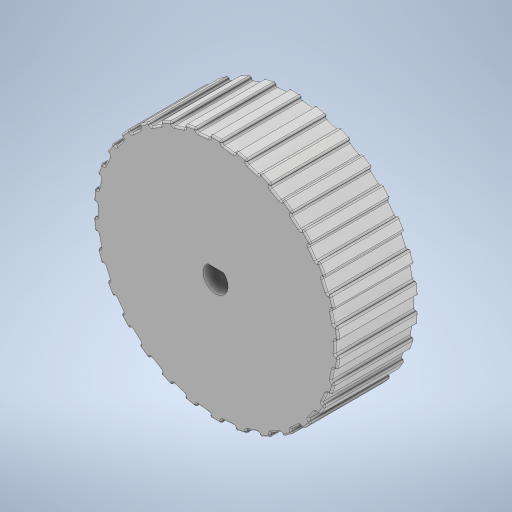
# Autodesk Inventor part: Tyre
Saved by Autodesk Inventor 2024 (Build 280153000, 153)
## iProperties
Created: 2024-04-29
Part Number: Tyre
Material: Generic
Document SubType Name: Modeling
Designer: Hitesh
Density: 1 g/cm^3
Appearance: Default
Author: Hitesh
Autodesk Inventor part; units mm, degrees
ref_plane "YZ Plane" through (0, 0, 0) normal (1, 0, 0) x (0, 1, 0)
ref_plane "XZ Plane" through (0, 0, 0) normal (0, 1, 0) x (-1, 0, 0)
ref_plane "XY Plane" through (0, 0, 0) normal (0, 0, 1) x (1, 0, 0)
sketch "Sketch1" plane through (0, 0, 0) normal (0, 0, 1) x (1, 0, 0)
  circle A0 centre (0, 0) radius 15.2 construction
  circle A1 centre (0, 0) radius 14.75
  circle A2 centre (0, 0) radius 13.5
  spline S0 degree 4 poles (-9.3055, 9.7805) (-7.3263, 12.0552) (-5.2624, 11.3174) (-0.0971, 11.8986) (3.041, 8.7469) (5.0437, 5.9417) (3.2663, 3.137) (1.327, 1.688) knots 0 0 0 0 0 0.374915 0.513644 0.64633 1 1 1 1 1
  circle A3 centre (0, 0) radius 2.1471
  spline S1 degree 4 poles (-11.2034, 7.5322) (-8.1625, 9.7041) (-7.2259, 9.5039) (-2.5238, 11.0895) (1.6832, 7.0671) (2.0649, 4.7541) (1.3, 2.8599) (0, 2.1471) knots 0 0 0 0 0 0.401494 0.546116 0.685045 1 1 1 1 1
  spline S2 degree 4 poles (-13.2771, 2.4429) (-13.0129, 5.4466) (-10.9095, 6.0628) (-7.0724, 9.5691) (-2.6811, 8.8638) (0.588, 7.7715) (0.7987, 4.4578) (0.0814, 2.1456) knots 0 0 0 0 0 0.374915 0.513644 0.64633 1 1 1 1 1
  spline S3 degree 4 poles (-13.4911, -0.4915) (-12.3075, 3.053) (-11.4322, 3.4416) (-8.5601, 7.4882) (-2.7922, 6.7067) (-1.1238, 5.0599) (-0.6293, 3.0778) (-1.2621, 1.7371) knots 0 0 0 0 0 0.401494 0.546116 0.685045 1 1 1 1 1
  spline S4 degree 4 poles (-12.1773, -5.8277) (-13.7291, -3.2424) (-12.3896, -1.5076) (-11.3462, 3.5845) (-7.3791, 5.5951) (-4.0923, 6.6329) (-1.9741, 4.0759) (-1.1953, 1.7837) knots 0 0 0 0 0 0.374915 0.513644 0.64633 1 1 1 1 1
  spline S5 degree 4 poles (-10.6256, -8.3274) (-11.7515, -4.7642) (-11.2717, -3.9354) (-11.3267, 1.0266) (-6.2011, 3.7846) (-3.8833, 3.433) (-2.3182, 2.1201) (-2.0421, 0.6635) knots 0 0 0 0 0 0.401494 0.546116 0.685045 1 1 1 1 1
  spline S6 degree 4 poles (-6.4262, -11.8724) (-9.2012, -10.693) (-9.1373, -8.5021) (-11.2862, -3.7692) (-9.2585, 0.1892) (-7.2094, 2.9608) (-3.9928, 2.1371) (-2.0154, 0.7404) knots 0 0 0 0 0 0.374915 0.513644 0.64633 1 1 1 1 1
  spline S7 degree 4 poles (-3.7016, -12.9826) (-6.7069, -10.7617) (-6.8059, -9.8091) (-9.7669, -5.8271) (-7.2413, -0.5831) (-5.1595, 0.4948) (-3.1216, 0.3526) (-2.0421, -0.6635) knots 0 0 0 0 0 0.401494 0.546116 0.685045 1 1 1 1 1
  spline S8 degree 4 poles (1.7795, -13.3822) (-1.1588, -14.0591) (-2.3948, -12.2491) (-6.9152, -9.6832) (-7.6015, -5.2889) (-7.5729, -1.8423) (-4.4864, -0.618) (-2.0657, -0.5856) knots 0 0 0 0 0 0.374915 0.513644 0.64633 1 1 1 1 1
  spline S9 degree 4 poles (4.6364, -12.6789) (0.8996, -12.6486) (0.2596, -11.9361) (-4.4765, -10.4551) (-5.5156, -4.728) (-4.4649, -2.6324) (-2.7327, -1.5496) (-1.2621, -1.7371) knots 0 0 0 0 0 0.401494 0.546116 0.685045 1 1 1 1 1
  spline S10 degree 4 poles (9.3055, -9.7805) (7.3263, -12.0552) (5.2624, -11.3174) (0.0971, -11.8986) (-3.041, -8.7469) (-5.0437, -5.9417) (-3.2663, -3.137) (-1.327, -1.688) knots 0 0 0 0 0 0.374915 0.513644 0.64633 1 1 1 1 1
  spline S11 degree 4 poles (11.2034, -7.5322) (8.1625, -9.7041) (7.2259, -9.5039) (2.5238, -11.0895) (-1.6832, -7.0671) (-2.0649, -4.7541) (-1.3, -2.8599) (0, -2.1471) knots 0 0 0 0 0 0.401494 0.546116 0.685045 1 1 1 1 1
  spline S12 degree 4 poles (13.2771, -2.4429) (13.0129, -5.4466) (10.9095, -6.0628) (7.0724, -9.5691) (2.6811, -8.8638) (-0.588, -7.7715) (-0.7987, -4.4578) (-0.0814, -2.1456) knots 0 0 0 0 0 0.374915 0.513644 0.64633 1 1 1 1 1
  spline S13 degree 4 poles (13.4911, 0.4915) (12.3075, -3.053) (11.4322, -3.4416) (8.5601, -7.4882) (2.7922, -6.7067) (1.1238, -5.0599) (0.6293, -3.0778) (1.2621, -1.7371) knots 0 0 0 0 0 0.401494 0.546116 0.685045 1 1 1 1 1
  spline S14 degree 4 poles (12.1773, 5.8277) (13.7291, 3.2424) (12.3896, 1.5076) (11.3462, -3.5845) (7.3791, -5.5951) (4.0923, -6.6329) (1.9741, -4.0759) (1.1953, -1.7837) knots 0 0 0 0 0 0.374915 0.513644 0.64633 1 1 1 1 1
  spline S15 degree 4 poles (10.6256, 8.3274) (11.7515, 4.7642) (11.2717, 3.9354) (11.3267, -1.0266) (6.2011, -3.7846) (3.8833, -3.433) (2.3182, -2.1201) (2.0421, -0.6635) knots 0 0 0 0 0 0.401494 0.546116 0.685045 1 1 1 1 1
  spline S16 degree 4 poles (6.4262, 11.8724) (9.2012, 10.693) (9.1373, 8.5021) (11.2862, 3.7692) (9.2585, -0.1892) (7.2094, -2.9608) (3.9928, -2.1371) (2.0154, -0.7404) knots 0 0 0 0 0 0.374915 0.513644 0.64633 1 1 1 1 1
  spline S17 degree 4 poles (3.7016, 12.9826) (6.7069, 10.7617) (6.8059, 9.8091) (9.7669, 5.8271) (7.2413, 0.5831) (5.1595, -0.4948) (3.1216, -0.3526) (2.0421, 0.6635) knots 0 0 0 0 0 0.401494 0.546116 0.685045 1 1 1 1 1
  spline S18 degree 4 poles (-1.7795, 13.3822) (1.1588, 14.0591) (2.3948, 12.2491) (6.9152, 9.6832) (7.6015, 5.2889) (7.5729, 1.8423) (4.4864, 0.618) (2.0657, 0.5856) knots 0 0 0 0 0 0.374915 0.513644 0.64633 1 1 1 1 1
  spline S19 degree 4 poles (-4.6364, 12.6789) (-0.8996, 12.6486) (-0.2596, 11.9361) (4.4765, 10.4551) (5.5156, 4.728) (4.4649, 2.6324) (2.7327, 1.5496) (1.2621, 1.7371) knots 0 0 0 0 0 0.401494 0.546116 0.685045 1 1 1 1 1
  line L0 (-0.715, 15.1832) -> (0.715, 15.1832)
  line L1 (0.715, 15.1832) -> (0.715, 14.7327)
  line L2 (-0.715, 14.7327) -> (-0.715, 15.1832)
  circle A4 centre (0, 0) radius 15.2 construction
  line L3 (-2.4574, 15) -> (-2.3638, 14.5594)
  line L4 (-3.8561, 14.7027) -> (-2.4574, 15)
  line L5 (-3.7624, 14.2621) -> (-3.8561, 14.7027)
  circle A5 centre (0, 0) radius 15.2 construction
  line L6 (-5.5224, 14.1613) -> (-5.3392, 13.7498)
  line L7 (-6.8287, 13.5797) -> (-5.5224, 14.1613)
  line L8 (-6.6455, 13.1682) -> (-6.8287, 13.5797)
  circle A6 centre (0, 0) radius 15.2 construction
  line L9 (-8.346, 12.7037) -> (-8.0812, 12.3392)
  line L10 (-9.5029, 11.8632) -> (-8.346, 12.7037)
  line L11 (-9.2381, 11.4987) -> (-9.5029, 11.8632)
  circle A7 centre (0, 0) radius 15.2 construction
  line L12 (-10.8049, 10.6909) -> (-10.4701, 10.3894)
  line L13 (-11.7617, 9.6282) -> (-10.8049, 10.6909)
  line L14 (-11.4269, 9.3268) -> (-11.7617, 9.6282)
  circle A8 centre (0, 0) radius 15.2 construction
  line L15 (-12.7915, 8.2108) -> (-12.4014, 7.9855)
  line L16 (-13.5065, 6.9724) -> (-12.7915, 8.2108)
  line L17 (-13.1163, 6.7472) -> (-13.5065, 6.9724)
  circle A9 centre (0, 0) radius 15.2 construction
  line L18 (-14.2191, 5.3718) -> (-13.7907, 5.2326)
  line L19 (-14.661, 4.0119) -> (-14.2191, 5.3718)
  line L20 (-14.2325, 3.8727) -> (-14.661, 4.0119)
  circle A10 centre (0, 0) radius 15.2 construction
  line L21 (-15.0253, 2.2981) -> (-14.5772, 2.251)
  line L22 (-15.1747, 0.876) -> (-15.0253, 2.2981)
  line L23 (-14.7267, 0.8289) -> (-15.1747, 0.876)
  circle A11 centre (0, 0) radius 15.2 construction
  line L24 (-15.1747, -0.876) -> (-14.7267, -0.8289)
  line L25 (-15.0253, -2.2981) -> (-15.1747, -0.876)
  line L26 (-14.5772, -2.251) -> (-15.0253, -2.2981)
  circle A12 centre (0, 0) radius 15.2 construction
  line L27 (-14.661, -4.0119) -> (-14.2325, -3.8727)
  line L28 (-14.2191, -5.3718) -> (-14.661, -4.0119)
  line L29 (-13.7907, -5.2326) -> (-14.2191, -5.3718)
  circle A13 centre (0, 0) radius 15.2 construction
  line L30 (-13.5065, -6.9724) -> (-13.1163, -6.7472)
  line L31 (-12.7915, -8.2108) -> (-13.5065, -6.9724)
  line L32 (-12.4014, -7.9855) -> (-12.7915, -8.2108)
  circle A14 centre (0, 0) radius 15.2 construction
  line L33 (-11.7617, -9.6282) -> (-11.4269, -9.3268)
  line L34 (-10.8049, -10.6909) -> (-11.7617, -9.6282)
  line L35 (-10.4701, -10.3894) -> (-10.8049, -10.6909)
  circle A15 centre (0, 0) radius 15.2 construction
  line L36 (-9.5029, -11.8632) -> (-9.2381, -11.4987)
  line L37 (-8.346, -12.7037) -> (-9.5029, -11.8632)
  line L38 (-8.0812, -12.3392) -> (-8.346, -12.7037)
  circle A16 centre (0, 0) radius 15.2 construction
  line L39 (-6.8287, -13.5797) -> (-6.6455, -13.1682)
  line L40 (-5.5224, -14.1613) -> (-6.8287, -13.5797)
  line L41 (-5.3392, -13.7498) -> (-5.5224, -14.1613)
  circle A17 centre (0, 0) radius 15.2 construction
  line L42 (-3.8561, -14.7027) -> (-3.7624, -14.2621)
  line L43 (-2.4574, -15) -> (-3.8561, -14.7027)
  line L44 (-2.3638, -14.5594) -> (-2.4574, -15)
  circle A18 centre (0, 0) radius 15.2 construction
  line L45 (-0.715, -15.1832) -> (-0.715, -14.7327)
  line L46 (0.715, -15.1832) -> (-0.715, -15.1832)
  line L47 (0.715, -14.7327) -> (0.715, -15.1832)
  circle A19 centre (0, 0) radius 15.2 construction
  line L48 (2.4574, -15) -> (2.3638, -14.5594)
  line L49 (3.8561, -14.7027) -> (2.4574, -15)
  line L50 (3.7624, -14.2621) -> (3.8561, -14.7027)
  circle A20 centre (0, 0) radius 15.2 construction
  line L51 (5.5224, -14.1613) -> (5.3392, -13.7498)
  line L52 (6.8287, -13.5797) -> (5.5224, -14.1613)
  line L53 (6.6455, -13.1682) -> (6.8287, -13.5797)
  circle A21 centre (0, 0) radius 15.2 construction
  line L54 (8.346, -12.7037) -> (8.0812, -12.3392)
  line L55 (9.5029, -11.8632) -> (8.346, -12.7037)
  line L56 (9.2381, -11.4987) -> (9.5029, -11.8632)
  circle A22 centre (0, 0) radius 15.2 construction
  line L57 (10.8049, -10.6909) -> (10.4701, -10.3894)
  line L58 (11.7617, -9.6282) -> (10.8049, -10.6909)
  line L59 (11.4269, -9.3268) -> (11.7617, -9.6282)
  circle A23 centre (0, 0) radius 15.2 construction
  line L60 (12.7915, -8.2108) -> (12.4014, -7.9855)
  line L61 (13.5065, -6.9724) -> (12.7915, -8.2108)
  line L62 (13.1163, -6.7472) -> (13.5065, -6.9724)
  circle A24 centre (0, 0) radius 15.2 construction
  line L63 (14.2191, -5.3718) -> (13.7907, -5.2326)
  line L64 (14.661, -4.0119) -> (14.2191, -5.3718)
  line L65 (14.2325, -3.8727) -> (14.661, -4.0119)
  circle A25 centre (0, 0) radius 15.2 construction
  line L66 (15.0253, -2.2981) -> (14.5772, -2.251)
  line L67 (15.1747, -0.876) -> (15.0253, -2.2981)
  line L68 (14.7267, -0.8289) -> (15.1747, -0.876)
  circle A26 centre (0, 0) radius 15.2 construction
  line L69 (15.1747, 0.876) -> (14.7267, 0.8289)
  line L70 (15.0253, 2.2981) -> (15.1747, 0.876)
  line L71 (14.5772, 2.251) -> (15.0253, 2.2981)
  circle A27 centre (0, 0) radius 15.2 construction
  line L72 (14.661, 4.0119) -> (14.2325, 3.8727)
  line L73 (14.2191, 5.3718) -> (14.661, 4.0119)
  line L74 (13.7907, 5.2326) -> (14.2191, 5.3718)
  circle A28 centre (0, 0) radius 15.2 construction
  line L75 (13.5065, 6.9724) -> (13.1163, 6.7472)
  line L76 (12.7915, 8.2108) -> (13.5065, 6.9724)
  line L77 (12.4014, 7.9855) -> (12.7915, 8.2108)
  circle A29 centre (0, 0) radius 15.2 construction
  line L78 (11.7617, 9.6282) -> (11.4269, 9.3268)
  line L79 (10.8049, 10.6909) -> (11.7617, 9.6282)
  line L80 (10.4701, 10.3894) -> (10.8049, 10.6909)
  circle A30 centre (0, 0) radius 15.2 construction
  line L81 (9.5029, 11.8632) -> (9.2381, 11.4987)
  line L82 (8.346, 12.7037) -> (9.5029, 11.8632)
  line L83 (8.0812, 12.3392) -> (8.346, 12.7037)
  circle A31 centre (0, 0) radius 15.2 construction
  line L84 (6.8287, 13.5797) -> (6.6455, 13.1682)
  line L85 (5.5224, 14.1613) -> (6.8287, 13.5797)
  line L86 (5.3392, 13.7498) -> (5.5224, 14.1613)
  circle A32 centre (0, 0) radius 15.2 construction
  line L87 (3.8561, 14.7027) -> (3.7624, 14.2621)
  line L88 (2.4574, 15) -> (3.8561, 14.7027)
  line L89 (2.3638, 14.5594) -> (2.4574, 15)
  point P0 (-6.1756, 11.4987)
  point P1 (-2.6972, 11.4438)
  point P2 (0.5481, 10.7598)
  point P3 (2.3826, 9.3005)
  point P4 (3.7011, 7.2393)
  point P5 (3.7427, 4.7755)
  point P6 (-7.424, 9.5544)
  point P7 (-4.8478, 9.9833)
  point P8 (-1.5394, 9.5539)
  point P9 (0.8289, 7.5318)
  point P10 (1.6333, 5.5146)
  point P11 (1.3948, 3.6994)
  point P12 (-5.881, 9.0271)
  point P13 (-3.5391, 8.9247)
  point P14 (-11.7549, 5.6728)
  point P15 (-8.9086, 7.6728)
  point P16 (-1.2609, 8.0322)
  point P17 (0.2209, 6.0634)
  point P18 (-6.861, 6.8244)
  point P19 (-3.7565, 6.5805)
  point P20 (-11.6221, 3.366)
  point P21 (-9.79, 5.2272)
  point P22 (-1.92, 5.4214)
  point P23 (-1.046, 3.8127)
  point P24 (-10.0638, 3.8463)
  point P25 (-8.109, 5.14)
  point P26 (-12.8443, -2.32)
  point P27 (-11.7172, 0.9711)
  point P28 (-5.7413, 5.7571)
  point P29 (-3.3852, 5.0353)
  point P30 (-9.562, 1.4883)
  point P31 (-6.907, 3.1157)
  point P32 (-11.3809, -4.1081)
  point P33 (-10.9928, -1.5255)
  point P34 (-4.7399, 3.2575)
  point P35 (-3.0873, 2.4697)
  point P36 (-10.4026, -2.8037)
  point P37 (-9.5816, -0.608)
  point P38 (-9.0276, -9.4266)
  point P39 (-10.0502, -6.1015)
  point P40 (-8.0287, 1.2829)
  point P41 (-5.6984, 2.0838)
  point P42 (-8.6106, -4.4164)
  point P43 (-7.4193, -1.5392)
  point P44 (-6.7927, -10.0131)
  point P45 (-7.9967, -7.6955)
  point P46 (-5.7494, -0.1507)
  point P47 (-3.9493, 0.1833)
  point P48 (-6.7679, -8.3827)
  point P49 (-7.3943, -6.1238)
  point P50 (-1.7627, -12.9326)
  point P51 (-4.5444, -10.8436)
  point P52 (-7.2494, -3.6813)
  point P53 (-5.8349, -1.6636)
  point P54 (-4.3702, -8.6341)
  point P55 (-5.0976, -5.6062)
  point P56 (0.3902, -12.0934)
  point P57 (-1.9461, -10.9261)
  point P58 (-4.5627, -3.5013)
  point P59 (-3.3028, -2.173)
  point P60 (-0.5481, -10.7598)
  point P61 (-2.3826, -9.3005)
  point P62 (6.1756, -11.4987)
  point P63 (2.6972, -11.4438)
  point P64 (-3.7011, -7.2393)
  point P65 (-3.7427, -4.7755)
  point P66 (1.5394, -9.5539)
  point P67 (-0.8289, -7.5318)
  point P68 (7.424, -9.5544)
  point P69 (4.8478, -9.9833)
  point P70 (-1.6333, -5.5146)
  point P71 (-1.3948, -3.6994)
  point P72 (5.881, -9.0271)
  point P73 (3.5391, -8.9247)
  point P74 (11.7549, -5.6728)
  point P75 (8.9086, -7.6728)
  point P76 (1.2609, -8.0322)
  point P77 (-0.2209, -6.0634)
  point P78 (6.861, -6.8244)
  point P79 (3.7565, -6.5805)
  point P80 (11.6221, -3.366)
  point P81 (9.79, -5.2272)
  point P82 (1.92, -5.4214)
  point P83 (1.046, -3.8127)
  point P84 (10.0638, -3.8463)
  point P85 (8.109, -5.14)
  point P86 (12.8443, 2.32)
  point P87 (11.7172, -0.9711)
  point P88 (5.7413, -5.7571)
  point P89 (3.3852, -5.0353)
  point P90 (9.562, -1.4883)
  point P91 (6.907, -3.1157)
  point P92 (11.3809, 4.1081)
  point P93 (10.9928, 1.5255)
  point P94 (4.7399, -3.2575)
  point P95 (3.0873, -2.4697)
  point P96 (10.4026, 2.8037)
  point P97 (9.5816, 0.608)
  point P98 (9.0276, 9.4266)
  point P99 (10.0502, 6.1015)
  point P100 (8.0287, -1.2829)
  point P101 (5.6984, -2.0838)
  point P102 (8.6106, 4.4164)
  point P103 (7.4193, 1.5392)
  point P104 (6.7927, 10.0131)
  point P105 (7.9967, 7.6955)
  point P106 (5.7494, 0.1507)
  point P107 (3.9493, -0.1833)
  point P108 (6.7679, 8.3827)
  point P109 (7.3943, 6.1238)
  point P110 (1.7627, 12.9326)
  point P111 (4.5444, 10.8436)
  point P112 (7.2494, 3.6813)
  point P113 (5.8349, 1.6636)
  point P114 (4.3702, 8.6341)
  point P115 (5.0976, 5.6062)
  point P116 (-0.3902, 12.0934)
  point P117 (1.9461, 10.9261)
  point P118 (4.5627, 3.5013)
  point P119 (3.3028, 2.173)
  point P120 (-4.6364, 12.6789)
  point P121 (1.2621, 1.7371)
  point P122 (-13.4911, -0.4915)
  point P123 (-1.2621, 1.7371)
  point P124 (-1.1953, 1.7837)
  point P125 (-12.1773, -5.8277)
  point P126 (-3.7016, -12.9826)
  point P127 (-2.0421, -0.6635)
  point P128 (-2.0657, -0.5856)
  point P129 (1.7795, -13.3822)
  point P130 (11.2034, -7.5322)
  point P131 (0, -2.1471)
  point P132 (-0.0814, -2.1456)
  point P133 (13.2771, -2.4429)
  point P134 (10.6256, 8.3274)
  point P135 (2.0421, -0.6635)
  point P136 (2.0154, -0.7404)
  point P137 (6.4262, 11.8724)
  point P138 (3.7016, 12.9826)
  point P139 (2.0421, 0.6635)
  point P140 (2.0657, 0.5856)
  point P141 (-1.7795, 13.3822)
  point P142 (13.4911, 0.4915)
  point P143 (1.2621, -1.7371)
  point P144 (1.1953, -1.7837)
  point P145 (12.1773, 5.8277)
  point P146 (4.6364, -12.6789)
  point P147 (-1.2621, -1.7371)
  point P148 (-1.327, -1.688)
  point P149 (9.3055, -9.7805)
  point P150 (-2.0421, 0.6635)
  point P151 (-2.0154, 0.7404)
  point P152 (-6.4262, -11.8724)
  point P153 (0.0814, 2.1456)
  point P154 (-13.2771, 2.4429)
  point P155 (1.3757, 1.7246)
  point P156 (-7.7747, 11.0365)
  point P157 (-12.8988, -3.9837)
  point P158 (-1.2151, 1.8413)
  point P159 (-2.1267, -0.5866)
  point P160 (-0.1972, -13.4986)
  point P161 (-0.0993, -2.2039)
  point P162 (12.7769, -4.3588)
  point P163 (2.0653, -0.7754)
  point P164 (8.0938, 10.8046)
  point P165 (2.1267, 0.5866)
  point P166 (0.1972, 13.4986)
  point P167 (1.2151, -1.8413)
  point P168 (12.8988, 3.9837)
  point P169 (-1.3757, -1.7246)
  point P170 (7.7747, -11.0365)
  point P171 (-2.0653, 0.7754)
  point P172 (-8.0938, -10.8046)
  point P173 (-12.7769, 4.3588)
  point P174 (0.0993, 2.2039)
  dimension "d0" = 30.4
  dimension "d1" = 29.5
  dimension "d2" = 27
  dimension "d3" = 4.2943
  dimension "d10" = 360
  dimension "d14" = 360
  constraints: 180 end point, 4 coincident, 2 point on circle, 1 centre point, 1 horizontal, 1 parallel, 1 perpendicular, 709 other
  measures "d3" diameter of A3
extrude "Extrusion1" add sketch "Sketch1" along normal blind 10 contours A1 | A1 L71 L70 L69 | L68 L67 L66 A1 | A1 L74 L73 L72 | L65 L64 L63 A1 | A1 L77 L76 L75 | L62 L61 L60 A1 | A1 L80 L79 L78 | L59 L58 L57 A1 | A1 L83 L82 L81 | L56 L55 L54 A1 | A1 L86 L85 L84 | L53 L52 L51 A1 | A1 L89 L88 L87 | L50 L49 L48 A1 | A1 L2 L0 L1 | L47 L46 L45 A1 | A1 L5 L4 L3 | L44 L43 L42 A1 | A1 L8 L7 L6 | L41 L40 L39 A1 | A1 L11 L10 L9 | L38 L37 L36 A1 | A1 L14 L13 L12 | L35 L34 L33 A1 | A1 L17 L16 L15 | L32 L31 L30 A1 | A1 L20 L19 L18 | L29 L28 L27 A1 | A1 L23 L22 L21 | L26 L25 L24 A1 | A2 S12 S11 A3 S14 S13 | S13 S14 A2 | S12 A2 | S14 S13 A3 S16 S15 A2 | A2 S14 | S14 A3 S13 | A2 S11 S12 | A3 | A2 S10 S9 A3 S12 S11 | S12 A3 S11 | S15 S16 A2 | A3 S15 S16 | S10 A2 | S16 S15 A3 S18 S17 A2 | A2 S16 | A2 S9 S10 | S9 S10 A3 | A2 S8 S7 A3 S10 S9 | S17 S18 A2 | A3 S17 S18 | S8 A2 | S7 S8 A3 | S18 S17 A3 S0 S19 A2 | A2 S18 | A2 S7 S8 | S8 S7 A2 S6 S5 A3 | A3 S19 S0 | S5 S6 A3 | S19 S0 A2 | S19 A3 S2 S1 A2 S0 | S6 A2 | S6 S5 A2 S4 S3 A3 | S6 A2 S5 | A2 S0 | A3 S1 S2 | S3 S4 A3 | A3 S4 S3 A2 S2 S1 | S2 A2 S1 | S4 A2 S3 | S4 A2 | A2 S2
fillet "Fillet1" radius 0.2 360 edges at (-15.1747, -0.876, 5) (-14.9507, -0.8525, 10) (-14.9507, -0.8525, 0) (-14.7267, 0.8289, 5) (-14.75, 0, 10) (-14.75, 0, 0) (-14.9507, 0.8525, 10) (-14.8012, 2.2746, 10) (-15.1, 1.5871, 10) (-14.4277, 3.0667, 10) (-15.1747, 0.876, 5) (-14.9507, 0.8525, 0) (-14.5772, 2.251, 5) (-14.8012, 2.2746, 0) (-15.0253, 2.2981, 5) (-15.1, 1.5871, 0) (-14.2325, 3.8727, 5) (-14.4277, 3.0667, 0) (-14.7267, -0.8289, 5) (-14.4468, 3.9423, 10) (-13.4748, 5.9994, 10) (-12.5965, 8.0981, 10) (-13.149, 7.5916, 10) (-12.5965, 8.0981, 0) (-11.5943, 9.4775, 0) (-10.6375, 10.5401, 0) (-11.2833, 10.1595, 0) (-9.3705, 11.681, 0) (-9.8697, 10.9614, 0) (-8.2136, 12.5215, 0) (-11.5943, 9.4775, 10) (-11.7617, 9.6282, 5) (-10.4701, 10.3894, 5) (-7.375, 12.7739, 0) (-10.8049, 10.6909, 5) (-10.6375, 10.5401, 10) (-11.2833, 10.1595, 10) (-9.2381, 11.4987, 5) (-9.8697, 10.9614, 10) (-9.3705, 11.681, 10) (-8.0812, 12.3392, 5) (-9.5029, 11.8632, 5) (-6.6455, 13.1682, 5) (-8.2136, 12.5215, 10) (-7.375, 12.7739, 10) (-8.9244, 12.2834, 10) (-8.346, 12.7037, 5) (-8.9244, 12.2834, 0) (-14.8012, -2.2746, 10) (-15.0253, -2.2981, 5) (-15.1, -1.5871, 0) (-14.0049, 5.3022, 10) (-14.4401, 4.6919, 10) (-13.3114, 6.8598, 10) (-14.661, 4.0119, 5) (-14.4468, 3.9423, 0) (-13.7907, 5.2326, 5) (-14.2191, 5.3718, 5) (-14.0049, 5.3022, 0) (-14.4401, 4.6919, 0) (-13.1163, 6.7472, 5) (-11.933, 8.6698, 10) (-13.4748, 5.9994, 0) (-13.5065, 6.9724, 5) (-13.3114, 6.8598, 0) (-12.4014, 7.9855, 5) (-12.7915, 8.2108, 5) (-11.4269, 9.3268, 5) (-11.933, 8.6698, 0) (-13.149, 7.5916, 0) (-15.1, -1.5871, 10) (-8.9244, -12.2834, 10) (-8.2136, -12.5215, 10) (-9.3705, -11.681, 10) (-7.375, -12.7739, 10) (-6.7371, -13.3739, 10) (-6.6455, -13.1682, 5) (-9.8697, -10.9614, 10) (-6.8287, -13.5797, 5) (-8.0812, -12.3392, 5) (-8.346, -12.7037, 5) (-8.2136, -12.5215, 0) (-7.375, -12.7739, 0) (-9.2381, -11.4987, 5) (-8.9244, -12.2834, 0) (-14.4277, -3.0667, 10) (-14.4401, -4.6919, 10) (-14.4468, -3.9423, 10) (-14.2325, -3.8727, 5) (-14.5772, -2.251, 5) (-14.661, -4.0119, 5) (-14.4277, -3.0667, 0) (-14.8012, -2.2746, 0) (-14.4468, -3.9423, 0) (-6.7371, -13.3739, 0) (10.4701, 10.3894, 5) (9.8697, 10.9614, 10) (9.8697, 10.9614, 0) (9.2381, 11.4987, 5) (9.3705, 11.681, 10) (9.3705, 11.681, 0) (9.5029, 11.8632, 5) (8.9244, 12.2834, 10) (8.9244, 12.2834, 0) (11.2833, 10.1595, 10) (11.2833, 10.1595, 0) (11.7617, 9.6282, 5) (10.8049, 10.6909, 5) (13.1163, 6.7472, 5) (11.5943, 9.4775, 10) (11.4269, 9.3268, 5) (10.6375, 10.5401, 0) (10.6375, 10.5401, 10) (11.933, 8.6698, 0) (11.933, 8.6698, 10) (12.4014, 7.9855, 5) (12.7915, 8.2108, 5) (12.5965, 8.0981, 0) (12.5965, 8.0981, 10) (-3.8093, 14.4824, 10) (-3.8093, 14.4824, 0) (-3.7624, 14.2621, 5) (-4.558, 14.0281, 10) (-4.558, 14.0281, 0) (-5.3392, 13.7498, 5) (-5.4308, 13.9555, 10) (-5.4308, 13.9555, 0) (-5.5224, 14.1613, 5) (-6.1756, 13.8705, 10) (-6.1756, 13.8705, 0) (-6.8287, 13.5797, 5) (-6.7371, 13.3739, 10) (-6.7371, 13.3739, 0) (0.715, -14.9579, 10) (0.715, -15.1832, 5) (0, -15.1832, 10) (0, -15.1832, 0) (13.7907, 5.2326, 5) (13.4748, 5.9994, 10) (13.4748, 5.9994, 0) (13.3114, 6.8598, 10) (13.3114, 6.8598, 0) (13.5065, 6.9724, 5) (13.149, 7.5916, 10) (13.149, 7.5916, 0) (14.7267, 0.8289, 5) (15.0253, 2.2981, 5) (14.8012, 2.2746, 10) (14.9507, 0.8525, 10) (15.1747, 0.876, 5) (15.1, 1.5871, 10) (14.75, 0, 0) (14.8012, 2.2746, 0) (15.1, 1.5871, 0) (14.9507, 0.8525, 0) (13.5065, -6.9724, 5) (13.3114, -6.8598, 10) (14.5772, 2.251, 5) (14.4277, 3.0667, 10) (14.4277, 3.0667, 0) (14.2325, 3.8727, 5) (14.2191, 5.3718, 5) (14.0049, 5.3022, 0) (14.4468, 3.9423, 0) (14.661, 4.0119, 5) (14.4401, 4.6919, 0) (14.0049, 5.3022, 10) (14.4401, 4.6919, 10) (14.4468, 3.9423, 10) (8.0812, -12.3392, 5) (9.5029, -11.8632, 5) (9.3705, -11.681, 10) (11.5943, -9.4775, 10) (11.4269, -9.3268, 5) (11.5943, -9.4775, 0) (10.4701, -10.3894, 5) (10.6375, -10.5401, 0) (9.8697, -10.9614, 10) (9.2381, -11.4987, 5) (9.8697, -10.9614, 0) (12.4014, -7.9855, 5) (11.933, -8.6698, 0) (12.5965, -8.0981, 10) (12.5965, -8.0981, 0) (9.3705, -11.681, 0) (13.4748, -5.9994, 10) (14.0049, -5.3022, 10) (14.4401, -4.6919, 10) (14.4468, -3.9423, 10) (13.1163, -6.7472, 5) (13.4748, -5.9994, 0) (14.4277, -3.0667, 10) (13.7907, -5.2326, 5) (14.8012, -2.2746, 10) (14.2191, -5.3718, 5) (14.0049, -5.3022, 0) (14.4401, -4.6919, 0) (14.2325, -3.8727, 5) (15.1, -1.5871, 10) (14.9507, -0.8525, 10) (14.4468, -3.9423, 0) (14.75, 0, 10) (14.4277, -3.0667, 0) (14.5772, -2.251, 5) (15.0253, -2.2981, 5) (14.8012, -2.2746, 0) (14.7267, -0.8289, 5) (15.1, -1.5871, 0) (15.1747, -0.876, 5) (14.9507, -0.8525, 0) (14.661, -4.0119, 5) (10.6375, -10.5401, 10) (11.7617, -9.6282, 5) (13.3114, -6.8598, 0) (12.7915, -8.2108, 5) (13.149, -7.5916, 10) (13.149, -7.5916, 0) (11.933, -8.6698, 10) (11.2833, -10.1595, 10) (10.8049, -10.6909, 5) (11.2833, -10.1595, 0) (6.6455, -13.1682, 5) (7.375, -12.7739, 10) (7.375, -12.7739, 0) (8.2136, -12.5215, 10) (8.2136, -12.5215, 0) (8.346, -12.7037, 5) (8.9244, -12.2834, 10) (8.9244, -12.2834, 0) (6.1756, -13.8705, 10) (6.7371, -13.3739, 10) (-1.5418, -14.6692, 10) (-0.715, -14.9579, 10) (-2.4106, -14.7797, 10) (-3.1568, -14.8514, 10) (-3.8093, -14.4824, 10) (-4.558, -14.0281, 10) (-5.4308, -13.9555, 10) (-6.1756, -13.8705, 10) (-0.715, -14.9579, 0) (-0.715, -15.1832, 5) (-1.5418, -14.6692, 0) (-0.715, -14.7327, 5) (-2.3638, -14.5594, 5) (-2.4106, -14.7797, 0) (-2.4574, -15, 5) (-3.1568, -14.8514, 0) (-3.8561, -14.7027, 5) (-3.8093, -14.4824, 0) (-3.7624, -14.2621, 5) (-4.558, -14.0281, 0) (-5.3392, -13.7498, 5) (-5.4308, -13.9555, 0) (-6.1756, -13.8705, 0) (-5.5224, -14.1613, 5) (3.7624, -14.2621, 5) (4.558, -14.0281, 10) (4.558, -14.0281, 0) (5.3392, -13.7498, 5) (5.5224, -14.1613, 5) (5.4308, -13.9555, 10) (5.4308, -13.9555, 0) (6.8287, -13.5797, 5) (6.1756, -13.8705, 0) (6.7371, -13.3739, 0) (-12.4014, -7.9855, 5) (-11.933, -8.6698, 10) (-11.933, -8.6698, 0) (-11.4269, -9.3268, 5) (-11.5943, -9.4775, 10) (-11.5943, -9.4775, 0) (-13.1163, -6.7472, 5) (-13.3114, -6.8598, 10) (-13.3114, -6.8598, 0) (-13.5065, -6.9724, 5) (-13.149, -7.5916, 10) (-11.7617, -9.6282, 5) (-11.2833, -10.1595, 10) (-10.8049, -10.6909, 5) (-10.6375, -10.5401, 10) (-10.6375, -10.5401, 0) (-11.2833, -10.1595, 0) (-10.4701, -10.3894, 5) (-12.7915, -8.2108, 5) (-12.5965, -8.0981, 10) (-13.7907, -5.2326, 5) (-13.4748, -5.9994, 10) (-14.4401, -4.6919, 0) (-14.0049, -5.3022, 10) (-14.2191, -5.3718, 5) (-9.5029, -11.8632, 5) (-13.4748, -5.9994, 0) (-14.0049, -5.3022, 0) (-9.3705, -11.681, 0) (-12.5965, -8.0981, 0) (-13.149, -7.5916, 0) (-9.8697, -10.9614, 0) (11.5943, 9.4775, 0) (3.8093, -14.4824, 10) (3.8093, -14.4824, 0) (3.8561, -14.7027, 5) (2.3638, -14.5594, 5) (2.4574, -15, 5) (3.1568, -14.8514, 10) (3.1568, -14.8514, 0) (2.4106, -14.7797, 10) (2.4106, -14.7797, 0) (1.5418, -14.6692, 10) (1.5418, -14.6692, 0) (0.715, -14.7327, 5) (0.715, -14.9579, 0) (-0.715, 14.7327, 5) (-0.715, 15.1832, 5) (-0.715, 14.9579, 0) (-1.5418, 14.6692, 10) (-1.5418, 14.6692, 0) (-2.3638, 14.5594, 5) (-2.4106, 14.7797, 0) (-2.4574, 15, 5) (-3.8561, 14.7027, 5) (-3.1568, 14.8514, 10) (-3.1568, 14.8514, 0) (3.7624, 14.2621, 5) (3.8093, 14.4824, 10) (3.8093, 14.4824, 0) (3.8561, 14.7027, 5) (3.1568, 14.8514, 10) (0, 15.1832, 0) (0.715, 14.9579, 10) (0.715, 14.9579, 0) (0.715, 15.1832, 5) (0.715, 14.7327, 5) (1.5418, 14.6692, 0) (2.4574, 15, 5) (2.4106, 14.7797, 0) (3.1568, 14.8514, 0) (2.3638, 14.5594, 5) (2.4106, 14.7797, 10) (-2.4106, 14.7797, 10) (-0.715, 14.9579, 10) (8.346, 12.7037, 5) (8.2136, 12.5215, 10) (8.2136, 12.5215, 0) (8.0812, 12.3392, 5) (7.375, 12.7739, 10) (7.375, 12.7739, 0) (6.6455, 13.1682, 5) (6.7371, 13.3739, 10) (6.7371, 13.3739, 0) (6.8287, 13.5797, 5) (6.1756, 13.8705, 10) (6.1756, 13.8705, 0) (5.5224, 14.1613, 5) (5.4308, 13.9555, 10) (5.4308, 13.9555, 0) (5.3392, 13.7498, 5) (4.558, 14.0281, 10) (4.558, 14.0281, 0) (1.5418, 14.6692, 10) (0, 15.1832, 10)
sketch "Sketch2" plane through (0, 0, 10) normal (0, 0, 1) x (1, 0, 0)
  circle A0 centre (0, 0) radius 1.55
  line L0 (0.9811, 1.2) -> (-0.9811, 1.2)
  dimension "d19" = 3.1
  dimension "d20" = 1.2
  constraints: 2 end point, 2 point on circle, 1 centre point, 1 coincident, 1 horizontal
  measures "d19" diameter of A0
  measures "d20" distance from line of A0.centre L0
extrude "Extrusion2" cut sketch "Sketch2" against normal through all contours A0 L0 picked at (0.4298, 0.1662)
body "Solid1"
